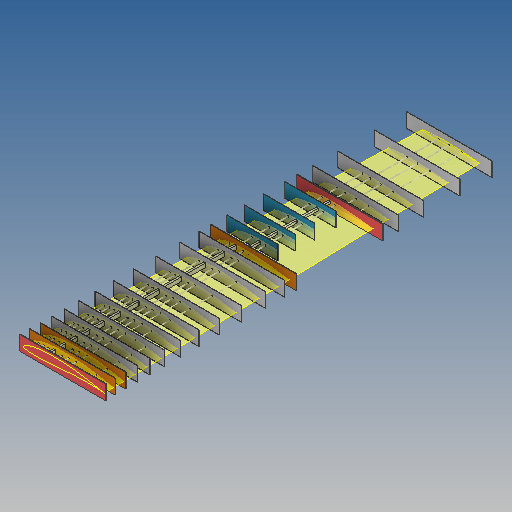
# Autodesk Inventor part: Skrzydlo-420-300_3
Saved by Autodesk Inventor 2025.3 (Build 293356000, 356)
## iProperties
Created: 2025-01-29
Part Number: Skrzydlo-420-300_3
Material: Generic
Document SubType Name: Modeling
Designer: abc
Density: 1 g/cm^3
Appearance: Default
Author: abc
Autodesk Inventor part; units mm, degrees
sketch "Sketch1" plane through (0, 0, 0) normal (0, 0, 1) x (1, 0, 0)
  spline S0 degree 4 poles (0, 0) (-0.0523, 1.5196) (0.9899, 3.3219) (3.3662, 5.7571) (7.4491, 8.7939) (11.4523, 11.1827) (16.3142, 13.5682) (21.9841, 15.9708) (28.4682, 18.2885) (35.7189, 20.5444) (43.7182, 22.6212) (52.4233, 24.6557) (61.8064, 26.4768) (71.8146, 28.2168) (82.4229, 29.6603) (93.5674, 30.997) (105.2206, 32.0121) (117.3167, 32.8919) (129.8101, 33.4333) (142.6447, 33.8358) (155.7703, 33.9067) (169.1229, 33.8197) (182.6579, 33.4298) (196.3035, 32.8776) (210.0076, 32.048) (223.7135, 31.1086) (237.358, 29.982) (250.8931, 28.7152) (264.2432, 27.2628) (277.3669, 25.693) (290.1984, 23.9721) (302.6861, 22.1554) (314.7783, 20.2541) (326.4226, 18.308) (337.5611, 16.3308) (348.1584, 14.4042) (358.1626, 12.5214) (367.5365, 10.7483) (376.2349, 9.0423) (384.2173, 7.4669) (391.4542, 5.9943) (397.9224, 4.6901) (403.5698, 3.5116) (408.4089, 2.5191) (412.3586, 1.65) (416.1486, 0.9157) (418.3641, 0.0679) (419.7505, 0.2661) (420, 0) knots 0 0 0 0 0 0.028631 0.042045 0.056882 0.073015 0.090316 0.108693 0.128061 0.148347 0.169479 0.191391 0.214021 0.237302 0.261176 0.285584 0.310468 0.335774 0.361446 0.387428 0.413669 0.440114 0.466707 0.493395 0.520121 0.54683 0.573467 0.599976 0.626301 0.652383 0.678166 0.70359 0.728591 0.753104 0.777061 0.800392 0.823025 0.844883 0.865887 0.885953 0.904983 0.922873 0.939498 0.954712 0.968322 0.980022 1 1 1 1 1
  spline S1 degree 4 poles (0, 0) (-0.0231, -1.1764) (1.0348, -2.6663) (3.4146, -4.3486) (7.5325, -5.7224) (11.5345, -6.8239) (16.3986, -7.651) (22.0573, -8.4955) (28.5347, -9.1134) (35.7773, -9.6929) (43.7636, -10.1004) (52.4654, -10.4462) (61.8408, -10.5642) (71.8489, -10.6444) (82.4489, -10.4598) (93.5932, -10.2593) (105.2392, -9.7632) (117.3349, -9.2335) (129.8221, -8.4314) (142.655, -7.5632) (155.7744, -6.4762) (169.124, -5.365) (182.653, -4.1055) (196.2961, -2.9035) (209.9969, -1.633) (223.7011, -0.4719) (237.3411, 0.7014) (250.8744, 1.6955) (264.2231, 2.6128) (277.3468, 3.3129) (290.1794, 3.8875) (302.6685, 4.3011) (314.7629, 4.5738) (326.41, 4.6991) (337.5534, 4.6986) (348.1532, 4.5361) (358.1607, 4.2949) (367.5341, 3.929) (376.2347, 3.516) (384.217, 3.0329) (391.4561, 2.5359) (397.9231, 2.0239) (403.5704, 1.5131) (408.4071, 1.0677) (412.3535, 0.5774) (416.1389, 0.3403) (418.3766, -0.0639) (419.7272, 0.0767) (420, 0) knots 0 0 0 0 0 0.02621 0.038778 0.052822 0.068275 0.085052 0.103045 0.12215 0.142278 0.163342 0.18526 0.20796 0.231369 0.25542 0.280048 0.305191 0.330786 0.356772 0.383089 0.409677 0.436476 0.463422 0.490457 0.517517 0.544546 0.571481 0.598262 0.624832 0.651129 0.677098 0.702679 0.727812 0.752435 0.776484 0.799894 0.822598 0.844521 0.865587 0.88571 0.904796 0.922742 0.939419 0.954674 0.968314 0.980048 1 1 1 1 1
  point P0 (419.5506, 0.1596)
  point P1 (418.2024, 0.3192)
  point P2 (415.9638, 0.8484)
  point P3 (412.8432, 1.5666)
  point P4 (408.8574, 2.4108)
  point P5 (404.0148, 3.423)
  point P6 (398.3448, 4.5948)
  point P7 (391.8642, 5.9136)
  point P8 (384.6066, 7.3794)
  point P9 (376.6056, 8.967)
  point P10 (367.8864, 10.668)
  point P11 (358.491, 12.4572)
  point P12 (348.4614, 14.3346)
  point P13 (337.8396, 16.2708)
  point P14 (326.6718, 18.2406)
  point P15 (315, 20.1936)
  point P16 (302.8788, 22.0962)
  point P17 (290.3628, 23.919)
  point P18 (277.5024, 25.6368)
  point P19 (264.3522, 27.2202)
  point P20 (250.971, 28.665)
  point P21 (237.4092, 29.946)
  point P22 (223.734, 31.0674)
  point P23 (210, 32.025)
  point P24 (196.266, 32.823)
  point P25 (182.5908, 33.3984)
  point P26 (169.029, 33.7596)
  point P27 (155.6478, 33.873)
  point P28 (142.4976, 33.7638)
  point P29 (129.6372, 33.3942)
  point P30 (117.1212, 32.8062)
  point P31 (105, 31.9578)
  point P32 (93.3282, 30.8952)
  point P33 (82.1604, 29.589)
  point P34 (71.5386, 28.0938)
  point P35 (61.509, 26.3802)
  point P36 (52.1136, 24.5154)
  point P37 (43.3944, 22.4952)
  point P38 (35.3934, 20.37)
  point P39 (28.1358, 18.1104)
  point P40 (21.6552, 15.7584)
  point P41 (15.9852, 13.3434)
  point P42 (11.1426, 10.9158)
  point P43 (7.1568, 8.4882)
  point P44 (4.0362, 6.1278)
  point P45 (1.7976, 3.969)
  point P46 (0.4494, 2.0244)
  point P47 (0.4494, -1.5414)
  point P48 (1.7976, -3.0072)
  point P49 (4.0362, -4.3806)
  point P50 (7.1568, -5.5608)
  point P51 (11.1426, -6.6402)
  point P52 (15.9852, -7.56)
  point P53 (21.6552, -8.379)
  point P54 (28.1358, -9.0552)
  point P55 (35.3934, -9.6222)
  point P56 (43.3944, -10.0632)
  point P57 (52.1136, -10.3866)
  point P58 (61.509, -10.5504)
  point P59 (71.5386, -10.5924)
  point P60 (82.1604, -10.4622)
  point P61 (93.3282, -10.2102)
  point P62 (105, -9.7692)
  point P63 (117.1212, -9.1938)
  point P64 (129.6372, -8.4336)
  point P65 (142.4976, -7.5348)
  point P66 (155.6478, -6.4848)
  point P67 (169.029, -5.3466)
  point P68 (182.5908, -4.1244)
  point P69 (196.266, -2.8938)
  point P70 (210, -1.6548)
  point P71 (223.734, -0.4662)
  point P72 (237.4092, 0.672)
  point P73 (250.971, 1.6884)
  point P74 (264.3522, 2.5788)
  point P75 (277.5024, 3.297)
  point P76 (290.3628, 3.864)
  point P77 (302.8788, 4.2798)
  point P78 (315, 4.5486)
  point P79 (326.6718, 4.6746)
  point P80 (337.8396, 4.662)
  point P81 (348.4614, 4.5108)
  point P82 (358.491, 4.2546)
  point P83 (367.8864, 3.8976)
  point P84 (376.6056, 3.4734)
  point P85 (384.6066, 2.9946)
  point P86 (391.8642, 2.4906)
  point P87 (398.3448, 1.974)
  point P88 (404.0148, 1.47)
  point P89 (408.8574, 0.9912)
  point P90 (412.8432, 0.5754)
  point P91 (415.9638, 0.2856)
  point P92 (418.2024, 0.0672)
  point P93 (419.5506, 0.0336)
  constraints: 98 other
ref_plane "Work Plane0" through (0, 0, -2008) normal (0, 0, 1) x (1, 0, 0)
sketch "Sketch2" plane through (0, 0, -2008) normal (0, 0, 1) x (1, 0, 0)
  spline S0 degree 4 poles (60, 0) (60.0066, 0.6561) (60.9154, 1.2788) (62.5875, 2.1359) (65.4118, 3.1676) (68.2515, 4.0135) (71.7124, 4.8585) (75.7526, 5.7136) (80.3757, 6.5383) (85.549, 7.3423) (91.254, 8.0822) (97.4694, 8.8082) (104.1663, 9.4577) (111.3142, 10.0788) (118.8866, 10.5938) (126.8457, 11.071) (135.1655, 11.4332) (143.8041, 11.7473) (152.725, 11.9405) (161.891, 12.0842) (171.2645, 12.1095) (180.8005, 12.0785) (190.4672, 11.9393) (200.2127, 11.7421) (210.0014, 11.4459) (219.7903, 11.1104) (229.5357, 10.7081) (239.2024, 10.2558) (248.7379, 9.7371) (258.1111, 9.1766) (267.2765, 8.562) (276.1964, 7.9133) (284.8343, 7.2342) (293.1525, 6.5391) (301.1106, 5.8328) (308.6809, 5.1447) (315.828, 4.4721) (322.5232, 3.839) (328.7372, 3.2296) (334.4389, 2.6669) (339.6092, 2.1409) (344.2288, 1.6752) (348.2631, 1.2543) (351.7185, 0.8999) (354.5407, 0.5895) (357.2435, 0.3275) (358.8414, 0.0235) (359.8086, 0.096) (360, 0) knots 0 0 0 0 0 0.023861 0.036167 0.050199 0.065751 0.082655 0.100781 0.120016 0.140266 0.16144 0.18346 0.206251 0.22974 0.253861 0.278548 0.303738 0.329369 0.355381 0.381714 0.40831 0.435111 0.46206 0.489098 0.516166 0.543209 0.570169 0.596987 0.623604 0.649962 0.676002 0.701664 0.726884 0.751598 0.77574 0.799242 0.822034 0.844039 0.86518 0.885371 0.904516 0.922512 0.939231 0.954524 0.968198 0.979963 1 1 1 1 1
  spline S1 degree 4 poles (60, 0) (60.0425, -0.5302) (60.9706, -1.0234) (62.6294, -1.5939) (65.4367, -2.0489) (68.271, -2.4418) (71.731, -2.733) (75.7676, -3.0352) (80.3888, -3.2549) (85.5602, -3.462) (91.2625, -3.6073) (97.4772, -3.7308) (104.1726, -3.7729) (111.3204, -3.8016) (118.8913, -3.7356) (126.8503, -3.664) (135.1689, -3.4869) (143.8074, -3.2978) (152.7272, -3.0113) (161.8929, -2.7013) (171.2653, -2.313) (180.8007, -1.9162) (190.4663, -1.4662) (200.2114, -1.037) (209.9994, -0.5831) (219.7881, -0.1684) (229.5326, 0.2506) (239.199, 0.6056) (248.7343, 0.9332) (258.1074, 1.1832) (267.2731, 1.3884) (276.1932, 1.5361) (284.8315, 1.6335) (293.1502, 1.6782) (301.1092, 1.6781) (308.6799, 1.62) (315.8276, 1.5339) (322.5227, 1.4033) (328.7372, 1.2558) (334.4388, 1.0832) (339.6095, 0.9057) (344.2289, 0.7229) (348.2632, 0.5405) (351.7181, 0.3814) (354.5397, 0.2062) (357.2417, 0.1215) (358.8436, -0.0229) (359.8042, 0.0274) (360, 0) knots 0 0 0 0 0 0.02263 0.034657 0.048458 0.063825 0.080596 0.098631 0.117811 0.138034 0.159207 0.181245 0.204072 0.227613 0.251798 0.276561 0.301837 0.327563 0.353676 0.380115 0.406821 0.433734 0.460794 0.487942 0.515118 0.542264 0.569321 0.59623 0.622932 0.649366 0.675474 0.701197 0.72647 0.751232 0.775417 0.798958 0.821786 0.843826 0.864999 0.885221 0.904395 0.922419 0.939164 0.95448 0.968172 0.979955 1 1 1 1 1
  point P0 (0, 0)
  point P1 (0, 0)
  point P2 (60.321, -0.5505)
  point P3 (61.284, -1.074)
  point P4 (62.883, -1.5645)
  point P5 (65.112, -1.986)
  point P6 (67.959, -2.3715)
  point P7 (71.418, -2.7)
  point P8 (75.468, -2.9925)
  point P9 (80.097, -3.234)
  point P10 (85.281, -3.4365)
  point P11 (90.996, -3.594)
  point P12 (97.224, -3.7095)
  point P13 (103.935, -3.768)
  point P14 (111.099, -3.783)
  point P15 (118.686, -3.7365)
  point P16 (126.663, -3.6465)
  point P17 (135, -3.489)
  point P18 (143.658, -3.2835)
  point P19 (152.598, -3.012)
  point P20 (161.784, -2.691)
  point P21 (171.177, -2.316)
  point P22 (180.735, -1.9095)
  point P23 (190.422, -1.473)
  point P24 (200.19, -1.0335)
  point P25 (210, -0.591)
  point P26 (219.81, -0.1665)
  point P27 (229.578, 0.24)
  point P28 (239.265, 0.603)
  point P29 (248.823, 0.921)
  point P30 (258.216, 1.1775)
  point P31 (267.402, 1.38)
  point P32 (276.342, 1.5285)
  point P33 (285, 1.6245)
  point P34 (293.337, 1.6695)
  point P35 (301.314, 1.665)
  point P36 (308.901, 1.611)
  point P37 (316.065, 1.5195)
  point P38 (322.776, 1.392)
  point P39 (329.004, 1.2405)
  point P40 (334.719, 1.0695)
  point P41 (339.903, 0.8895)
  point P42 (344.532, 0.705)
  point P43 (348.582, 0.525)
  point P44 (352.041, 0.354)
  point P45 (354.888, 0.2055)
  point P46 (357.117, 0.102)
  point P47 (358.716, 0.024)
  point P48 (359.679, 0.012)
  point P49 (359.679, 0.057)
  point P50 (358.716, 0.114)
  point P51 (357.117, 0.303)
  point P52 (354.888, 0.5595)
  point P53 (352.041, 0.861)
  point P54 (348.582, 1.2225)
  point P55 (344.532, 1.641)
  point P56 (339.903, 2.112)
  point P57 (334.719, 2.6355)
  point P58 (329.004, 3.2025)
  point P59 (322.776, 3.81)
  point P60 (316.065, 4.449)
  point P61 (308.901, 5.1195)
  point P62 (301.314, 5.811)
  point P63 (293.337, 6.5145)
  point P64 (285, 7.212)
  point P65 (276.342, 7.8915)
  point P66 (267.402, 8.5425)
  point P67 (258.216, 9.156)
  point P68 (248.823, 9.7215)
  point P69 (239.265, 10.2375)
  point P70 (229.578, 10.695)
  point P71 (219.81, 11.0955)
  point P72 (210, 11.4375)
  point P73 (200.19, 11.7225)
  point P74 (190.422, 11.928)
  point P75 (180.735, 12.057)
  point P76 (171.177, 12.0975)
  point P77 (161.784, 12.0585)
  point P78 (152.598, 11.9265)
  point P79 (143.658, 11.7165)
  point P80 (135, 11.4135)
  point P81 (126.663, 11.034)
  point P82 (118.686, 10.5675)
  point P83 (111.099, 10.0335)
  point P84 (103.935, 9.4215)
  point P85 (97.224, 8.7555)
  point P86 (90.996, 8.034)
  point P87 (85.281, 7.275)
  point P88 (80.097, 6.468)
  point P89 (75.468, 5.628)
  point P90 (71.418, 4.7655)
  point P91 (67.959, 3.8985)
  point P92 (65.112, 3.0315)
  point P93 (62.883, 2.1885)
  point P94 (61.284, 1.4175)
  point P95 (60.321, 0.723)
  constraints: 98 other
surface_loft "LoftSrf1"
sketch "Sketch3" plane through (0, 0, 0) normal (0, 0, 1) x (1, 0, 0)
  line L0 (-18.8418, -30.5799) -> (426.1582, -30.5799)
  line L1 (426.1582, -30.5799) -> (426.1582, 44.4201)
  line L2 (426.1582, 44.4201) -> (-18.8418, 44.4201)
  line L3 (-18.8418, 44.4201) -> (-18.8418, -30.5799)
  point P0 (0, 0)
  dimension "d5" = 445
  dimension "d6" = 75
  constraints: 8 end point, 2 parallel, 1 horizontal, 1 perpendicular
  measures "d5" distance of L2.end L1.end
  measures "d6" distance of L1.end L0.end
extrude "c0" add sketch "Sketch3" against normal blind 4
ref_plane "Work Plane2" through (0, 0, -50) normal (0, 0, 1) x (1, 0, 0)
ref_plane "Work Plane3" through (0, 0, -105) normal (0, 0, 1) x (1, 0, 0)
ref_plane "Work Plane4" through (0, 0, -165) normal (0, 0, 1) x (1, 0, 0)
ref_plane "Work Plane5" through (0, 0, -230) normal (0, 0, 1) x (1, 0, 0)
ref_plane "Work Plane6" through (0, 0, -305) normal (0, 0, 1) x (1, 0, 0)
ref_plane "Work Plane7" through (0, 0, -390) normal (0, 0, 1) x (1, 0, 0)
ref_plane "Work Plane8" through (0, 0, -485) normal (0, 0, 1) x (1, 0, 0)
ref_plane "Work Plane9" through (0, 0, -590) normal (0, 0, 1) x (1, 0, 0)
ref_plane "Work Plane10" through (0, 0, -705) normal (0, 0, 1) x (1, 0, 0)
ref_plane "Work Plane11" through (0, 0, -830) normal (0, 0, 1) x (1, 0, 0)
ref_plane "Work Plane12" through (0, 0, -930) normal (0, 0, 1) x (1, 0, 0)
ref_plane "Work Plane13" through (0, 0, -990) normal (0, 0, 1) x (1, 0, 0)
ref_plane "Work Plane14" through (0, 0, -1075) normal (0, 0, 1) x (1, 0, 0)
ref_plane "Work Plane15" through (0, 0, -1165) normal (0, 0, 1) x (1, 0, 0)
ref_plane "Work Plane16" through (0, 0, -1265) normal (0, 0, 1) x (1, 0, 0)
ref_plane "Work Plane17" through (0, 0, -1375) normal (0, 0, 1) x (1, 0, 0)
ref_plane "Work Plane18" through (0, 0, -1438) normal (0, 0, 1) x (1, 0, 0)
ref_plane "Work Plane19" through (0, 0, -1520) normal (0, 0, 1) x (1, 0, 0)
ref_plane "Work Plane20" through (0, 0, -1650) normal (0, 0, 1) x (1, 0, 0)
ref_plane "Work Plane21" through (0, 0, -1840) normal (0, 0, 1) x (1, 0, 0)
ref_plane "Work Plane22" through (0, 0, -2006) normal (0, 0, 1) x (1, 0, 0)
sketch "Sketch4" plane through (0, 0, -50) normal (0, 0, 1) x (1, 0, 0)
  line L0 (-18.8418, -30.5799) -> (426.1582, -30.5799)
  line L1 (426.1582, -30.5799) -> (426.1582, 44.4201)
  line L2 (426.1582, 44.4201) -> (-18.8418, 44.4201)
  line L3 (-18.8418, 44.4201) -> (-18.8418, -30.5799)
  point P0 (0, 0)
  point P1 (0, 0)
  dimension "d30" = 445
  dimension "d31" = 75
  constraints: 8 end point, 2 parallel, 1 horizontal, 1 perpendicular
  measures "d30" distance of L2.end L1.end
  measures "d31" distance of L1.end L0.end
extrude "c1" add sketch "Sketch4" against normal blind 3
sketch "Sketch5" plane through (0, 0, -105) normal (0, 0, 1) x (1, 0, 0)
  line L0 (-18.8418, -30.5799) -> (426.1582, -30.5799)
  line L1 (426.1582, -30.5799) -> (426.1582, 44.4201)
  line L2 (426.1582, 44.4201) -> (-18.8418, 44.4201)
  line L3 (-18.8418, 44.4201) -> (-18.8418, -30.5799)
  point P0 (0, 0)
  point P1 (0, 0)
  dimension "d34" = 445
  dimension "d35" = 75
  constraints: 8 end point, 2 parallel, 1 horizontal, 1 perpendicular
  measures "d34" distance of L2.end L1.end
  measures "d35" distance of L1.end L0.end
extrude "c2" add sketch "Sketch5" against normal blind 3
sketch "Sketch6" plane through (0, 0, -165) normal (0, 0, 1) x (1, 0, 0)
  line L0 (-18.8418, -30.5799) -> (426.1582, -30.5799)
  line L1 (426.1582, -30.5799) -> (426.1582, 44.4201)
  line L2 (426.1582, 44.4201) -> (-18.8418, 44.4201)
  line L3 (-18.8418, 44.4201) -> (-18.8418, -30.5799)
  point P0 (0, 0)
  point P1 (0, 0)
  dimension "d38" = 445
  dimension "d39" = 75
  constraints: 8 end point, 2 parallel, 1 horizontal, 1 perpendicular
  measures "d38" distance of L2.end L1.end
  measures "d39" distance of L1.end L0.end
extrude "c3" add sketch "Sketch6" against normal blind 2
sketch "Sketch7" plane through (0, 0, -230) normal (0, 0, 1) x (1, 0, 0)
  line L0 (-18.8418, -30.5799) -> (426.1582, -30.5799)
  line L1 (426.1582, -30.5799) -> (426.1582, 44.4201)
  line L2 (426.1582, 44.4201) -> (-18.8418, 44.4201)
  line L3 (-18.8418, 44.4201) -> (-18.8418, -30.5799)
  point P0 (0, 0)
  point P1 (0, 0)
  dimension "d42" = 445
  dimension "d43" = 75
  constraints: 8 end point, 2 parallel, 1 horizontal, 1 perpendicular
  measures "d42" distance of L2.end L1.end
  measures "d43" distance of L1.end L0.end
extrude "c4" add sketch "Sketch7" against normal blind 2
sketch "Sketch8" plane through (0, 0, -305) normal (0, 0, 1) x (1, 0, 0)
  line L0 (-18.8418, -30.5799) -> (426.1582, -30.5799)
  line L1 (426.1582, -30.5799) -> (426.1582, 44.4201)
  line L2 (426.1582, 44.4201) -> (-18.8418, 44.4201)
  line L3 (-18.8418, 44.4201) -> (-18.8418, -30.5799)
  point P0 (0, 0)
  point P1 (0, 0)
  dimension "d46" = 445
  dimension "d47" = 75
  constraints: 8 end point, 2 parallel, 1 horizontal, 1 perpendicular
  measures "d46" distance of L2.end L1.end
  measures "d47" distance of L1.end L0.end
extrude "c5" add sketch "Sketch8" against normal blind 2
sketch "Sketch9" plane through (0, 0, -390) normal (0, 0, 1) x (1, 0, 0)
  line L0 (-18.8418, -30.5799) -> (426.1582, -30.5799)
  line L1 (426.1582, -30.5799) -> (426.1582, 44.4201)
  line L2 (426.1582, 44.4201) -> (-18.8418, 44.4201)
  line L3 (-18.8418, 44.4201) -> (-18.8418, -30.5799)
  point P0 (0, 0)
  point P1 (0, 0)
  dimension "d50" = 445
  dimension "d51" = 75
  constraints: 8 end point, 2 parallel, 1 horizontal, 1 perpendicular
  measures "d50" distance of L2.end L1.end
  measures "d51" distance of L1.end L0.end
extrude "c6" add sketch "Sketch9" against normal blind 2
sketch "Sketch10" plane through (0, 0, -485) normal (0, 0, 1) x (1, 0, 0)
  line L0 (-18.8418, -30.5799) -> (426.1582, -30.5799)
  line L1 (426.1582, -30.5799) -> (426.1582, 44.4201)
  line L2 (426.1582, 44.4201) -> (-18.8418, 44.4201)
  line L3 (-18.8418, 44.4201) -> (-18.8418, -30.5799)
  point P0 (0, 0)
  point P1 (0, 0)
  dimension "d54" = 445
  dimension "d55" = 75
  constraints: 8 end point, 2 parallel, 1 horizontal, 1 perpendicular
  measures "d54" distance of L2.end L1.end
  measures "d55" distance of L1.end L0.end
extrude "c7" add sketch "Sketch10" against normal blind 2
sketch "Sketch11" plane through (0, 0, -590) normal (0, 0, 1) x (1, 0, 0)
  line L0 (-18.8418, -30.5799) -> (426.1582, -30.5799)
  line L1 (426.1582, -30.5799) -> (426.1582, 44.4201)
  line L2 (426.1582, 44.4201) -> (-18.8418, 44.4201)
  line L3 (-18.8418, 44.4201) -> (-18.8418, -30.5799)
  point P0 (0, 0)
  point P1 (0, 0)
  dimension "d58" = 445
  dimension "d59" = 75
  constraints: 8 end point, 2 parallel, 1 horizontal, 1 perpendicular
  measures "d58" distance of L2.end L1.end
  measures "d59" distance of L1.end L0.end
extrude "c8" add sketch "Sketch11" against normal blind 2
sketch "Sketch12" plane through (0, 0, -705) normal (0, 0, 1) x (1, 0, 0)
  line L0 (-18.8418, -30.5799) -> (426.1582, -30.5799)
  line L1 (426.1582, -30.5799) -> (426.1582, 44.4201)
  line L2 (426.1582, 44.4201) -> (-18.8418, 44.4201)
  line L3 (-18.8418, 44.4201) -> (-18.8418, -30.5799)
  point P0 (0, 0)
  point P1 (0, 0)
  dimension "d62" = 445
  dimension "d63" = 75
  constraints: 8 end point, 2 parallel, 1 horizontal, 1 perpendicular
  measures "d62" distance of L2.end L1.end
  measures "d63" distance of L1.end L0.end
extrude "c9" add sketch "Sketch12" against normal blind 2
sketch "Sketch13" plane through (0, 0, -830) normal (0, 0, 1) x (1, 0, 0)
  line L0 (-18.8418, -30.5799) -> (426.1582, -30.5799)
  line L1 (426.1582, -30.5799) -> (426.1582, 44.4201)
  line L2 (426.1582, 44.4201) -> (-18.8418, 44.4201)
  line L3 (-18.8418, 44.4201) -> (-18.8418, -30.5799)
  point P0 (0, 0)
  point P1 (0, 0)
  dimension "d66" = 445
  dimension "d67" = 75
  constraints: 8 end point, 2 parallel, 1 horizontal, 1 perpendicular
  measures "d66" distance of L2.end L1.end
  measures "d67" distance of L1.end L0.end
extrude "c10" add sketch "Sketch13" against normal blind 2
sketch "Sketch14" plane through (0, 0, -930) normal (0, 0, 1) x (1, 0, 0)
  line L0 (-18.8418, -30.5799) -> (426.1582, -30.5799)
  line L1 (426.1582, -30.5799) -> (426.1582, 44.4201)
  line L2 (426.1582, 44.4201) -> (-18.8418, 44.4201)
  line L3 (-18.8418, 44.4201) -> (-18.8418, -30.5799)
  point P0 (0, 0)
  point P1 (0, 0)
  dimension "d70" = 445
  dimension "d71" = 75
  constraints: 8 end point, 2 parallel, 1 horizontal, 1 perpendicular
  measures "d70" distance of L2.end L1.end
  measures "d71" distance of L1.end L0.end
extrude "c11" add sketch "Sketch14" against normal blind 2
sketch "Sketch15" plane through (0, 0, -990) normal (0, 0, 1) x (1, 0, 0)
  line L0 (-18.8418, -30.5799) -> (426.1582, -30.5799)
  line L1 (426.1582, -30.5799) -> (426.1582, 44.4201)
  line L2 (426.1582, 44.4201) -> (-18.8418, 44.4201)
  line L3 (-18.8418, 44.4201) -> (-18.8418, -30.5799)
  point P0 (0, 0)
  point P1 (0, 0)
  dimension "d74" = 445
  dimension "d75" = 75
  constraints: 8 end point, 2 parallel, 1 horizontal, 1 perpendicular
  measures "d74" distance of L2.end L1.end
  measures "d75" distance of L1.end L0.end
extrude "c12" add sketch "Sketch15" against normal blind 3
sketch "Sketch16" plane through (0, 0, -1075) normal (0, 0, 1) x (1, 0, 0)
  line L0 (426.1582, 44.4201) -> (-18.8418, 44.4201) projected
  line L1 (426.1582, -30.5799) -> (-18.8418, -30.5799) projected
  line L2 (-18.8418, 44.4201) -> (246.1582, 44.4201)
  line L3 (246.1582, 44.4201) -> (246.1582, -30.5799)
  line L4 (246.1582, -30.5799) -> (-18.8418, -30.5799)
  line L5 (-18.8418, -30.5799) -> (-18.8418, 44.4201)
  point P0 (0, 0)
  dimension "d78" = 265
  constraints: 8 end point, 2 parallel, 1 horizontal, 1 perpendicular, 1 point on line
  measures "d78" distance of L3.end L4.end
extrude "c13K" add sketch "Sketch16" against normal blind 2
sketch "Sketch17" plane through (0, 0, -1165) normal (0, 0, 1) x (1, 0, 0)
  line L0 (-18.8418, 44.4201) -> (246.1582, 44.4201)
  line L1 (246.1582, 44.4201) -> (246.1582, -30.5799)
  line L2 (246.1582, -30.5799) -> (-18.8418, -30.5799)
  line L3 (-18.8418, -30.5799) -> (-18.8418, 44.4201)
  point P0 (0, 0)
  point P1 (0, 0)
  point P2 (-18.8418, -30.5799)
  dimension "d81" = 265
  constraints: 8 end point, 2 parallel, 1 horizontal, 1 perpendicular
  measures "d81" distance of L1.end L2.end
extrude "c14K" add sketch "Sketch17" against normal blind 2
sketch "Sketch18" plane through (0, 0, -1265) normal (0, 0, 1) x (1, 0, 0)
  line L0 (-18.8418, 44.4201) -> (246.1582, 44.4201)
  line L1 (246.1582, 44.4201) -> (246.1582, -30.5799)
  line L2 (246.1582, -30.5799) -> (-18.8418, -30.5799)
  line L3 (-18.8418, -30.5799) -> (-18.8418, 44.4201)
  point P0 (0, 0)
  point P1 (0, 0)
  point P2 (-18.8418, -30.5799)
  dimension "d84" = 265
  constraints: 8 end point, 2 parallel, 1 horizontal, 1 perpendicular
  measures "d84" distance of L1.end L2.end
extrude "c15K" add sketch "Sketch18" against normal blind 2
sketch "Sketch19" plane through (0, 0, -1375) normal (0, 0, 1) x (1, 0, 0)
  line L0 (-18.8418, 44.4201) -> (246.1582, 44.4201)
  line L1 (246.1582, 44.4201) -> (246.1582, -30.5799)
  line L2 (246.1582, -30.5799) -> (-18.8418, -30.5799)
  line L3 (-18.8418, -30.5799) -> (-18.8418, 44.4201)
  point P0 (0, 0)
  point P1 (0, 0)
  point P2 (-18.8418, -30.5799)
  dimension "d87" = 265
  constraints: 8 end point, 2 parallel, 1 horizontal, 1 perpendicular
  measures "d87" distance of L1.end L2.end
extrude "c16K" add sketch "Sketch19" against normal blind 2
sketch "Sketch20" plane through (0, 0, -1438) normal (0, 0, 1) x (1, 0, 0)
  line L0 (-18.8418, -30.5799) -> (426.1582, -30.5799)
  line L1 (426.1582, -30.5799) -> (426.1582, 44.4201)
  line L2 (426.1582, 44.4201) -> (-18.8418, 44.4201)
  line L3 (-18.8418, 44.4201) -> (-18.8418, -30.5799)
  point P0 (0, 0)
  point P1 (0, 0)
  point P2 (0, 0)
  dimension "d90" = 445
  dimension "d91" = 75
  constraints: 8 end point, 2 parallel, 1 horizontal, 1 perpendicular
  measures "d90" distance of L2.end L1.end
  measures "d91" distance of L1.end L0.end
extrude "c17" add sketch "Sketch20" against normal blind 4
sketch "Sketch21" plane through (0, 0, -1520) normal (0, 0, 1) x (1, 0, 0)
  line L0 (-18.8418, -30.5799) -> (426.1582, -30.5799)
  line L1 (426.1582, -30.5799) -> (426.1582, 44.4201)
  line L2 (426.1582, 44.4201) -> (-18.8418, 44.4201)
  line L3 (-18.8418, 44.4201) -> (-18.8418, -30.5799)
  point P0 (0, 0)
  point P1 (0, 0)
  point P2 (0, 0)
  dimension "d94" = 445
  dimension "d95" = 75
  constraints: 8 end point, 2 parallel, 1 horizontal, 1 perpendicular
  measures "d94" distance of L2.end L1.end
  measures "d95" distance of L1.end L0.end
extrude "c18" add sketch "Sketch21" against normal blind 2
sketch "Sketch22" plane through (0, 0, -1650) normal (0, 0, 1) x (1, 0, 0)
  line L0 (-18.8418, -30.5799) -> (426.1582, -30.5799)
  line L1 (426.1582, -30.5799) -> (426.1582, 44.4201)
  line L2 (426.1582, 44.4201) -> (-18.8418, 44.4201)
  line L3 (-18.8418, 44.4201) -> (-18.8418, -30.5799)
  point P0 (0, 0)
  point P1 (0, 0)
  point P2 (0, 0)
  dimension "d98" = 445
  dimension "d99" = 75
  constraints: 8 end point, 2 parallel, 1 horizontal, 1 perpendicular
  measures "d98" distance of L2.end L1.end
  measures "d99" distance of L1.end L0.end
extrude "c19" add sketch "Sketch22" against normal blind 2
sketch "Sketch23" plane through (0, 0, -1840) normal (0, 0, 1) x (1, 0, 0)
  line L0 (-18.8418, -30.5799) -> (426.1582, -30.5799)
  line L1 (426.1582, -30.5799) -> (426.1582, 44.4201)
  line L2 (426.1582, 44.4201) -> (-18.8418, 44.4201)
  line L3 (-18.8418, 44.4201) -> (-18.8418, -30.5799)
  point P0 (0, 0)
  point P1 (0, 0)
  point P2 (0, 0)
  dimension "d102" = 445
  dimension "d103" = 75
  constraints: 8 end point, 2 parallel, 1 horizontal, 1 perpendicular
  measures "d102" distance of L2.end L1.end
  measures "d103" distance of L1.end L0.end
extrude "c20" add sketch "Sketch23" against normal blind 2
sketch "Sketch24" plane through (0, 0, -2006) normal (0, 0, 1) x (1, 0, 0)
  line L0 (-18.8418, -30.5799) -> (426.1582, -30.5799)
  line L1 (426.1582, -30.5799) -> (426.1582, 44.4201)
  line L2 (426.1582, 44.4201) -> (-18.8418, 44.4201)
  line L3 (-18.8418, 44.4201) -> (-18.8418, -30.5799)
  point P0 (0, 0)
  point P1 (0, 0)
  point P2 (0, 0)
  dimension "d106" = 445
  dimension "d107" = 75
  constraints: 8 end point, 2 parallel, 1 horizontal, 1 perpendicular
  measures "d106" distance of L2.end L1.end
  measures "d107" distance of L1.end L0.end
extrude "c21" add sketch "Sketch24" against normal blind 2
sketch "Sketch26" plane through (0, 0, 0) normal (0, 0, 1) x (1, 0, 0)
  line L0 (105, -2) -> (115, -2)
  line L1 (115, -2) -> (115, 18)
  line L2 (115, 18) -> (105, 18)
  line L3 (105, 18) -> (105, -2)
  point P0 (0, 0)
  dimension "d112" = 10
  dimension "d113" = 20
  dimension "d114" = 105
  dimension "d115" = 18
  constraints: 8 end point, 2 parallel, 1 horizontal, 1 perpendicular
  measures "d112" distance of L2.end L1.end
  measures "d113" distance of L1.end L0.end
  measures "d114" distance from line of point (0, 0) L3
  measures "d115" distance from line of point (0, 0) L2
extrude "d1" add sketch "Sketch26" against normal up to surface (993 mm away)
sketch "Sketch27" plane through (0, 0, -993) normal (0, 0, -1) x (-1, 0, 0)
  line L0 (-155, 0) -> (-145, 0)
  line L1 (-145, 0) -> (-145, 12)
  line L2 (-145, 12) -> (-155, 12)
  line L3 (-155, 12) -> (-155, 0)
  line L4 (-105, 18) -> (-115, 18) projected
  line L5 (-115, 18) -> (-115, -2) projected
  point P0 (0, 0)
  point P1 (-115, 8)
  point P2 (-150, 0)
  dimension "d118" = 10
  dimension "d119" = 12
  dimension "d120" = 6
  dimension "d159" = 35
  constraints: 8 end point, 2 midpoint, 2 parallel, 1 horizontal, 1 perpendicular
  measures "d118" distance of L2.end L1.end
  measures "d119" distance of L1.end L0.end
  measures "d120" distance between parallel lines of L4 L2
  measures "d159" distance from line of L5 point (-150, 0)
extrude "d2" add sketch "Sketch27" along normal up to surface (449 mm away)
sketch "Sketch28" plane through (0, 0, 0) normal (0, 0, 1) x (1, 0, 0)
  circle A0 centre (80, 8) radius 3
  line L0 (105, 18) -> (105, -2) projected
  line L1 (115, 18) -> (105, 18) projected
  point P0 (0, 0)
  dimension "d124" = 6
  dimension "d125" = 25
  dimension "d126" = 10
  constraints: 1 centre point
  measures "d124" diameter of A0
  measures "d125" distance from line of L0 A0.centre
  measures "d126" distance from line of L1 A0.centre
extrude "p1" add sketch "Sketch28" against normal up to surface (993 mm away)
sketch "Sketch29" plane through (0, 0, 0) normal (0, 0, 1) x (1, 0, 0)
  circle A0 centre (55, 8) radius 3
  circle A1 centre (80, 8) radius 3 projected
  line L0 (115, 18) -> (105, 18) projected
  point P0 (0, 0)
  dimension "d129" = 6
  dimension "d130" = 25
  constraints: 1 centre point
  measures "d129" diameter of A0
  measures "d130" distance of A1.centre A0.centre
extrude "p2" add sketch "Sketch29" against normal up to surface (707 mm away) contours A0
sketch "Sketch30" plane through (0, 0, 0) normal (0, 0, 1) x (1, 0, 0)
  circle A0 centre (30.3221, 4) radius 3
  circle A1 centre (55, 8) radius 3 projected
  line L0 (105, -2) -> (115, -2) projected
  point P0 (0, 0)
  dimension "d134" = 6
  dimension "d135" = 25
  dimension "d148" = 6
  constraints: 1 centre point
  measures "d134" diameter of A0
  measures "d135" distance of A1.centre A0.centre
  measures "d148" distance from line of L0 A0.centre
extrude "p3" add sketch "Sketch30" against normal up to surface (392 mm away) contours A0
sketch "Sketch31" plane through (0, 0, 0) normal (0, 0, 1) x (1, 0, 0)
  circle A0 centre (150, 8) radius 3
  line L0 (115, -2) -> (115, 18) projected
  line L1 (115, 18) -> (105, 18) projected
  point P0 (0, 0)
  dimension "d138" = 6
  dimension "d139" = 35
  dimension "d140" = 10
  constraints: 1 centre point
  measures "d138" diameter of A0
  measures "d139" distance from line of L0 A0.centre
  measures "d140" distance from line of L1 A0.centre
extrude "p4" add sketch "Sketch31" against normal up to surface (993 mm away)
sketch "Sketch32" plane through (0, 0, 0) normal (0, 0, 1) x (1, 0, 0)
  circle A0 centre (184.4819, 14) radius 3
  line L0 (115, 18) -> (105, 18) projected
  circle A1 centre (150, 8) radius 3 projected
  point P0 (0, 0)
  dimension "d143" = 6
  dimension "d144" = 4
  dimension "d145" = 35
  constraints: 1 centre point
  measures "d143" diameter of A0
  measures "d144" distance from line of L0 A0.centre
  measures "d145" distance of A1.centre A0.centre
extrude "p5" add sketch "Sketch32" against normal up to surface (932 mm away) contours A0
sketch "Sketch33" plane through (0, 0, 0) normal (0, 0, 1) x (1, 0, 0)
  circle A0 centre (224.4819, 18) radius 2
  circle A1 centre (184.4819, 14) radius 3 projected
  line L0 (115, 18) -> (105, 18) projected
  point P0 (0, 0)
  dimension "d149" = 4
  dimension "d150" = 40
  dimension "d151" = 0
  constraints: 1 centre point
  measures "d149" diameter of A0
  measures "d150" horizontal distance of A1.centre A0.centre
  measures "d151" distance from line of L0 A0.centre
extrude "p6" add sketch "Sketch33" against normal up to surface (592 mm away) contours A0
sketch "Sketch34" plane through (0, 0, 0) normal (0, 0, 1) x (1, 0, 0)
  circle A0 centre (329.4819, 11) radius 2
  circle A1 centre (224.4819, 18) radius 2 projected
  line L0 (115, 18) -> (105, 18) projected
  point P0 (0, 0)
  dimension "d154" = 4
  dimension "d155" = 105
  dimension "d156" = 7
  constraints: 1 centre point
  measures "d154" diameter of A0
  measures "d155" horizontal distance of A1.centre A0.centre
  measures "d156" distance from line of L0 A0.centre
extrude "p7" add sketch "Sketch34" against normal up to surface (307 mm away) contours A0
sketch "Sketch35" plane through (0, 0, -305) normal (0, 0, 1) x (1, 0, 0)
  circle A0 centre (224.4819, 18) radius 2 projected
  circle A1 centre (274.4819, 12) radius 2
  point P0 (0, 0)
  dimension "d160" = 4
  dimension "d161" = 50
  dimension "d165" = 6
  constraints: 1 centre point
  measures "d160" diameter of A1
  measures "d161" horizontal distance of A0.centre A1.centre
  measures "d165" vertical distance of A0.centre A1.centre
extrude "p8" add sketch "Sketch35" against normal up to surface (527 mm away) contours A1
sketch "Sketch36" plane through (0, 0, -993) normal (0, 0, -1) x (-1, 0, 0)
  circle A0 centre (-110, 8) radius 3
  line L0 (-105, -2) -> (-105, 18) projected
  line L1 (-105, 18) -> (-115, 18) projected
  point P0 (0, 0)
  dimension "d166" = 6
  dimension "d167" = 5
  dimension "d168" = 10
  constraints: 1 centre point
  measures "d166" diameter of A0
  measures "d167" distance from line of L0 A0.centre
  measures "d168" distance from line of A0.centre L1
extrude "p9d1" add sketch "Sketch36" along normal up to surface (659 mm away)
sketch "Sketch37" plane through (0, 0, -1442) normal (0, 0, -1) x (-1, 0, 0)
  circle A0 centre (-150, 6) radius 3
  line L0 (-145, 0) -> (-145, 12) projected
  line L1 (-155, 0) -> (-145, 0) projected
  point P0 (0, 0)
  dimension "d171" = 6
  dimension "d172" = 5
  dimension "d173" = 6
  constraints: 1 centre point
  measures "d171" diameter of A0
  measures "d172" distance from line of L0 A0.centre
  measures "d173" distance from line of L1 A0.centre
extrude "p10d2" add sketch "Sketch37" along normal up to surface (566 mm away)
sketch "Sketch38" plane through (0, 0, -2008) normal (0, 0, -1) x (-1, 0, 0)
  circle A0 centre (-270, 5) radius 2
  line L0 (-155, 12) -> (-155, 0) projected
  line L1 (-155, 0) -> (-145, 0) projected
  point P0 (0, 0)
  dimension "d176" = 4
  dimension "d177" = 115
  dimension "d178" = 5
  constraints: 1 centre point
  measures "d176" diameter of A0
  measures "d177" distance from line of L0 A0.centre
  measures "d178" distance from line of L1 A0.centre
extrude "p11" add sketch "Sketch38" against normal up to surface (570 mm away)
sketch "Sketch39" plane through (0, 0, -1442) normal (0, 0, -1) x (-1, 0, 0)
  circle A0 centre (-150, 6) radius 3 projected
  circle A1 centre (-205, 6) radius 3
  line L0 (-145, 12) -> (-155, 12) projected
  point P0 (0, 0)
  dimension "d181" = 6
  dimension "d182" = 55
  dimension "d183" = 6
  constraints: 1 centre point
  measures "d181" diameter of A1
  measures "d182" distance of A0.centre A1.centre
  measures "d183" distance from line of L0 A1.centre
extrude "p12" add sketch "Sketch39" along normal up to surface (566 mm away) contours A1
sketch "Sketch41" plane through (0, 0, -990) normal (0, 0, 1) x (1, 0, 0)
  circle A0 centre (180, 6) radius 3
  circle A1 centre (150, 6) radius 3 projected
  point P0 (0, 0)
  dimension "d186" = 6
  dimension "d187" = 30
  dimension "d188" = 0
  constraints: 1 centre point
  measures "d186" diameter of A0
  measures "d187" distance of A1.centre A0.centre
  measures "d188" vertical distance of A1.centre A0.centre
extrude "p13K" add sketch "Sketch41" against normal up to surface (452 mm away) contours A0
body "Solid1"
body "Srf1"
